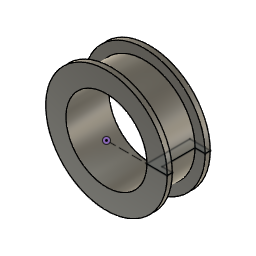
idler-pulley (Autodesk Fusion 360 design; units mm, degrees)
Autodesk Fusion 360 part; units mm, degrees
sketch "Sketch1" plane through (0, 0, 0) normal (0, 0, 1) x (1, 0, 0)
  line L0 (0, 0) -> (8, 0) construction
  line L1 (8, 0) -> (8, 8.5)
  line L2 (8, 8.5) -> (12, 8.5)
  line L3 (12, 8.5) -> (12, 7.5)
  line L4 (12, 7.5) -> (10, 7.5)
  line L5 (10, 7.5) -> (10, 1)
  line L6 (10, 1) -> (12, 1)
  line L7 (12, 1) -> (12, 0)
  line L8 (12, 0) -> (8, 0)
  dimension "d1" = 1
  dimension "d2" = 1
  dimension "d3" = 6.5
  dimension "d4" = 8
  dimension "d5" = 2
  dimension "d6" = 2
  constraint coincident L0.start origin
  constraint horizontal L0
  constraint perpendicular L0 L1
  constraint perpendicular L1 L2
  constraint perpendicular L2 L3
  constraint perpendicular L1 L4
  constraint perpendicular L4 L5
  constraint perpendicular L1 L6
  constraint perpendicular L4 L7
  constraint perpendicular L1 L8
  constraint collinear L3 L7
  measures "d1" distance of L2.end L3.end
  measures "d2" distance of L6.end L7.end
  measures "d3" distance of L4.end L5.end
  measures "d4" distance of L0.start L1
  measures "d5" distance of L3 L5
  measures "d6" distance of L1 L5
revolve "Revolve1" add sketch "Sketch1" angle 360 about axis through (0, 1.75, 0) along (0, 1, 0)
